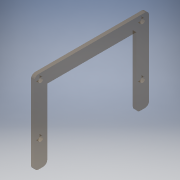
# Autodesk Inventor part: ArmSpacer
Saved by Autodesk Inventor 2019 (Build 230136000, 136)
## iProperties
Created: 2019-01-14
Part Number: ArmSpacer
Material: Polycarbonate, Smoke
Document SubType Name: Modeling
Designer: nxgam
Density: 1.2 g/cm^3
Appearance: Polycarbonate - Smoked
Author: nxgam
Autodesk Inventor part; units mm, degrees
ref_plane "YZ Plane" through (0, 0, 0) normal (1, 0, 0) x (0, 1, 0)
ref_plane "XZ Plane" through (0, 0, 0) normal (0, 1, 0) x (-1, 0, 0)
ref_plane "XY Plane" through (0, 0, 0) normal (0, 0, 1) x (1, 0, 0)
sketch "Sketch1" plane through (0, 0, 0) normal (1, 0, 0) x (0, 1, 0)
  line L0 (0, 45.72) -> (66.04, 45.72)
  line L1 (66.04, 45.72) -> (66.04, -45.72)
  line L2 (66.04, -45.72) -> (0, -45.72)
  line L3 (0, 35.56) -> (55.88, 35.56)
  line L4 (55.88, 35.56) -> (55.88, -35.56)
  line L5 (55.88, -35.56) -> (0, -35.56)
  line L6 (55.88, 35.56) -> (66.04, 45.72) construction
  line L7 (55.88, -35.56) -> (66.04, -45.72) construction
  line L8 (0, 45.72) -> (0, -45.72) construction
  line L9 (0, -45.72) -> (0, -35.56)
  line L10 (0, 35.56) -> (0, 45.72)
  point P0 (0, 0)
  point P1 (60.96, 40.64)
  point P2 (60.96, -40.64)
  point P3 (20.32, -40.64)
  point P4 (20.32, 40.64)
  point P5 (0, 0)
  dimension "d0" = 71.12
  dimension "d1" = 10.16
  dimension "d2" = 10.16
  dimension "d3" = 10.16
  dimension "d4" = 66.04
  dimension "d7" = 40.64
  constraints: 22 end point, 3 horizontal, 3 midpoint, 3 perpendicular, 2 collinear, 1 coincident, 1 parallel, 1 point on line, 2 other
  measures "d0" distance of L3.end L4.end
  measures "d1" distance between parallel lines of L2 L5
  measures "d2" distance between parallel lines of L0 L3
  measures "d3" distance between parallel lines of L1 L4
  measures "d4" distance of L1.end L2.end
  measures "d7" distance of point (60.96, -40.64) point (20.32, -40.64)
extrude "Extrusion2" add sketch "Sketch1" along normal blind 2.794
hole "Hole2" at (0, 60.96, 40.64) at (0, 60.96, -40.64) at (0, 20.32, -40.64) at (0, 20.32, 40.64) direction (1, 0, 0) diameter 4 end through all
fillet "Fillet1" radius 3.175 6 edges at (1.397, 0, -35.56) (1.397, 0, 35.56) (1.397, 0, -45.72) (1.397, 0, 45.72) (1.397, 66.04, 45.72) (1.397, 66.04, -45.72)
equation "\"d2\" = d1"
equation "\"d3\" = d2"
body "Solid1"
